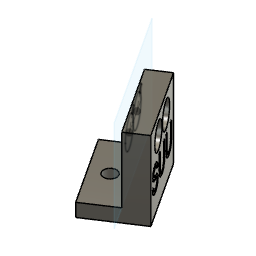
Diode Bracket v7 (Autodesk Fusion 360 design; units mm, degrees)
Autodesk Fusion 360 part; units mm, degrees
note: some values were not read from the file. Chosen so that the rebuilt part matches the saved one: which face or edge a step refers to. Set by a fixed rule: which sketch regions a step uses.
sketch "Sketch1" plane through (0, 0, 0) normal (0, 1, 0) x (1, 0, 0)
  line L0 (150.8044, 29.9826) -> (178.1974, -11.8459)
  circle A0 centre (169.8131, 12.5472) radius 2.08
  line L1 (150.8044, 29.9826) -> (168.1214, 41.3233)
  line L2 (168.1214, 41.3233) -> (195.5144, -0.5052)
  line L3 (178.1974, -11.8459) -> (195.5144, -0.5052)
  circle A1 centre (169.8131, 12.5472) radius 3.175
  circle A2 centre (169.8131, 12.5472) radius 2.5
  dimension "d32" = 5
  constraint concentric A0 A2
  measures "d32" diameter of A2
extrude "Extrude1" add sketch "Sketch1" along normal blind 5 contours L0 L1 L2 L3 | A1
sketch "Sketch2" plane through (0, 5, 0) normal (0, 1, 0) x (-1, 0, 0)
  line L0 (-150.8044, -29.9826) -> (-178.1974, 11.8459)
  line L1 (-178.1974, 11.8459) -> (-195.5144, 0.5052)
  line L2 (-195.5144, 0.5052) -> (-168.1214, -41.3233)
  line L3 (-168.1214, -41.3233) -> (-150.8044, -29.9826)
  line L4 (-161.4288, -36.9404) -> (-188.8218, 4.8881)
  line L5 (-169.8131, -12.5472) -> (-164.5009, -9.0683) construction
  line L6 (-169.8131, -12.5472) -> (-175.1253, -16.0261) construction
  circle A0 centre (-169.8131, -12.5472) radius 2.5
  constraint coincident L3 L4.start
  constraint coincident L1 L4.end
  constraint perpendicular L1 L4
  constraint midpoint L0 L5.end
  constraint midpoint L4 L6.end
  constraint equal L5 L6
extrude "Extrude2" add sketch "Sketch2" along normal blind 35 contours L1 L2 L3 L4
sketch "Sketch3" plane through (135.5953, 0, -88.7997) normal (0.83657, 0, -0.54786) x (-0.54786, 0, -0.83657)
  line L0 (-79.6052, 0) -> (-70.6052, 0)
  line L1 (-70.6052, 40) -> (-79.6052, 40)
  line L2 (-79.6052, 40) -> (-79.6052, 0)
  circle A0 centre (-77.45, 23) radius 4.75
  dimension "d5" = 23
  dimension "d17" = 9.5
  measures "d5" distance of L0 A0.centre
  measures "d17" diameter of A0
extrude "Extrude3" cut sketch "Sketch3" against normal up to surface (6.8 mm away)
sketch "Sketch4" plane through (135.5953, 0, -88.7997) normal (0.83657, 0, -0.54786) x (-0.54786, 0, -0.83657)
  line L0 (-94.469, 0) -> (-85.469, 0)
  line L1 (-85.469, 0) -> (-85.469, 40)
  line L2 (-85.469, 40) -> (-94.469, 40)
  circle A0 centre (-87.5449, 23) radius 4.75
  dimension "d8" = 23
  dimension "d18" = 9.5
  measures "d8" distance of L0 A0.centre
  measures "d18" diameter of A0
extrude "Extrude4" cut sketch "Sketch4" against normal up to surface (6.8 mm away)
extrude "Extrude5" cut 1 faces at (178.4607, 21.1568, -23.345) along direction (0.83657, 0, -0.54786) up to surface (1.2 mm away)
extrude "Extrude6" cut 1 faces at (182.6998, 20.6101, -16.872) along direction (0.83657, 0, -0.54786) up to surface (1.2 mm away)
sketch "Sketch5" plane through (136.5991, 0, -89.4571) normal (0.83657, 0, -0.54786) x (-0.54786, 0, -0.83657)
  circle A0 centre (-87.5449, 23) radius 4.75
  circle A1 centre (-77.45, 23) radius 4.75
  line L0 (-107.5371, 0) -> (-57.5371, 0)
  line L1 (-57.5371, 0) -> (-57.5371, 40)
  line L2 (-57.5371, 40) -> (-107.5371, 40)
  line L3 (-107.5371, 40) -> (-107.5371, 0)
  line L4 (-91.9862, 16.5574) -> (-107.5371, 16.5574)
  line L5 (-73.088, 12) -> (-57.5371, 12)
  line L6 (-95.1764, 7.1043) -> (-69.888, 7.1043) construction
  line L7 (-69.888, 7.1043) -> (-69.888, 19.6512) construction
  line L8 (-69.888, 19.6512) -> (-95.1764, 19.6512) construction
  line L9 (-95.1764, 19.6512) -> (-95.1764, 7.1043) construction
  dimension "d31" = 12
  text T0 "SUU" font "Arial" height 12.5469 align ink ink in box 0 x 0 at (-95.1664, 7.1243) x (1, 0) y (0, 1) spacing 1 height is em
  constraint coincident L3 L4.end
  constraint coincident L1 L5.end
  constraint horizontal L4
  constraint horizontal L5
  constraint equal L4 L5
  constraint perpendicular L6 L7
  constraint parallel L6 L8
  constraint parallel L7 L9
  measures "d31" vertical distance of L0.end L5.end
extrude "Extrude7" cut sketch "Sketch5" against normal blind 2 text T0
sketch "Sketch6" plane through (129.9066, 0, -85.0742) normal (-0.83657, 0, 0.54786) x (0.54786, 0, 0.83657)
  circle A0 centre (87.5449, 23) radius 4.75
  circle A1 centre (77.45, 23) radius 4.75
  line L0 (57.5371, 5) -> (107.5371, 5)
  line L1 (107.5371, 5) -> (107.5371, 40)
  line L2 (107.5371, 40) -> (57.5371, 40)
  line L3 (57.5371, 40) -> (57.5371, 5)
  circle A2 centre (77.45, 23) radius 5.25
  circle A3 centre (87.5449, 23) radius 5.25
  line L4 (74.3061, 27.2046) -> (73.2455, 26.1439)
  line L5 (73.2455, 26.1439) -> (71.5484, 27.841)
  line L6 (71.5484, 27.841) -> (72.6091, 28.9016)
  line L7 (72.6091, 28.9016) -> (74.3061, 27.2046)
  line L8 (84.401, 27.2046) -> (83.3403, 26.1439)
  line L9 (83.3403, 26.1439) -> (81.6433, 27.841)
  line L10 (81.6433, 27.841) -> (82.7039, 28.9016)
  line L11 (82.7039, 28.9016) -> (84.401, 27.2046)
  line L12 (77.45, 23) -> (72.0787, 28.3713) construction
  line L13 (87.5449, 23) -> (82.1736, 28.3713) construction
  line L14 (77.45, 23) -> (87.5449, 23) construction
  line L15 (77.45, 23) -> (72.0787, 23) construction
  line L16 (72.0787, 23) -> (72.0787, 28.3713) construction
  dimension "d19" = 10.5
  dimension "d20" = 10.5
  dimension "d23" = 1.5
  dimension "d24" = 1.5
  dimension "d25" = 2.4
  dimension "d27" = 2.4
  constraint concentric A1 A2
  constraint concentric A0 A3
  constraint perpendicular L4 L5
  constraint parallel L4 L6
  constraint parallel L5 L7
  constraint coincident A2 L4.end
  constraint coincident A2 L4.start
  constraint perpendicular L8 L9
  constraint parallel L8 L10
  constraint parallel L9 L11
  constraint coincident A3 L8.end
  constraint coincident A3 L8.start
  constraint coincident A1.centre A2.centre
  constraint midpoint L6 L12.end
  constraint perpendicular L6 L12
  constraint coincident A0.centre A3.centre
  constraint midpoint L10 L13.end
  constraint perpendicular L10 L13
  constraint parallel L12 L13
  constraint horizontal L15
  constraint perpendicular L15 L16
  constraint equal L15 L16
  measures "d19" diameter of A3
  measures "d20" diameter of A2
  measures "d23" distance of L5.end L6.end
  measures "d24" distance of L9.end L10.end
  measures "d25" distance of L4.start L6.end
  measures "d27" distance of L8.start L10.end
extrude "Extrude9" cut sketch "Sketch6" against normal blind 4.5 contours A2 A3 L4 | A2 L5 L6 L7 | A2 A3 L8 | A2 A3 | A3 L9 L10 L11
extrude "Extrude8" cut sketch "Sketch6" against normal blind 4.5 contours A2 L4 | A2 A3 L4 | A2 A3 L8 | A2 A3 | A3 L8
extrude "Extrude10" cut 1 faces at (172.7907, 40, -24.4585) along direction (0, -1, 0) blind 10
extrude "Extrude11" cut 1 faces at (165.8905, 11.6667, -39.8623) along direction (0.54786, 0, 0.83657) blind 10
extrude "Extrude12" cut 1 faces at (193.2835, 11.6667, 1.9662) along direction (-0.54786, 0, -0.83657) blind 10
